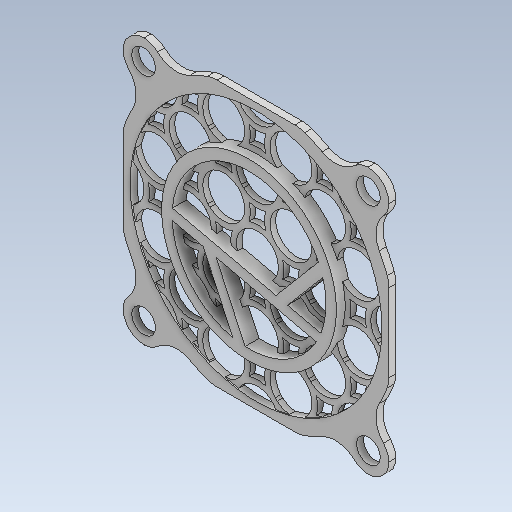
# Autodesk Inventor part: S Fan Cover
Saved by Autodesk Inventor 2022 (Build 260153000, 153)
## iProperties
Created: 2019-12-19
Part Number: S Fan Cover
Material: Generic
Document SubType Name: Modeling
Designer: pepd9
Density: 1 g/cm^3
Appearance: Default
Author: pepd9
Autodesk Inventor part; units mm, degrees
ref_plane "YZ Plane" through (0, 0, 0) normal (1, 0, 0) x (0, 1, 0)
ref_plane "XZ Plane" through (0, 0, 0) normal (0, 1, 0) x (-1, 0, 0)
ref_plane "XY Plane" through (0, 0, 0) normal (0, 0, 1) x (1, 0, 0)
sketch "Sketch1" plane through (0, 0, 0) normal (0, 0, 1) x (1, 0, 0)
  circle A0 centre (1.9624, -34.0934) radius 1.5 projected
  circle A1 centre (1.9624, -1.9624) radius 1.5 projected
  circle A2 centre (34.0934, -1.9624) radius 1.5 projected
  circle A3 centre (34.0934, -34.0934) radius 1.5 projected
  line L0 (1.9624, -34.0934) -> (34.0934, -1.9624)
  line L1 (37.0279, -37.0279) -> (-0.9721, -37.0279)
  line L2 (-0.9721, -37.0279) -> (-0.9721, 0.9721)
  line L3 (-0.9721, 0.9721) -> (37.0279, 0.9721)
  line L4 (37.0279, 0.9721) -> (37.0279, -37.0279)
  line L5 (37.0279, -37.0279) -> (-0.9721, 0.9721) construction
  line L6 (-0.9721, -37.0279) -> (37.0279, 0.9721) construction
  circle A4 centre (1.9624, -34.0934) radius 1.7
  circle A5 centre (34.0934, -34.0934) radius 1.7
  circle A6 centre (34.0934, -1.9624) radius 1.7
  circle A7 centre (1.9624, -1.9624) radius 1.7
  point P0 (0, 0)
  point P1 (18.0279, -18.0279)
  dimension "d0" = 38
  dimension "d1" = 38
  dimension "d5" = 0.2
  dimension "d6" = 0.2
  dimension "d7" = 0.2
  dimension "d8" = 0.2
  constraints: 14 end point, 4 centre point, 3 midpoint, 2 parallel, 1 horizontal, 1 perpendicular
  measures "d0" distance of L2.end L3.end
  measures "d1" distance of L1.end L2.end
  measures "d5" radial gap between concentric circles of A0 A4
  measures "d6" radial gap between concentric circles of A3 A5
  measures "d7" radial gap between concentric circles of A2 A6
  measures "d8" radial gap between concentric circles of A1 A7
extrude "Extrusion1" add sketch "Sketch1" along normal blind 1 contours L1 L2 L3 L4
fillet "Fillet1" radius 3 4 edges at (-0.9721, 0.9721, 0.5) (-0.9721, -37.0279, 0.5) (37.0279, -37.0279, 0.5) (37.0279, 0.9721, 0.5)
sketch "Sketch2" plane through (0, 0, 1) normal (0, 0, 1) x (1, 0, 0)
  arc A0 (37.0279, -2.0279) -> (34.0279, 0.9721) centre (34.0279, -2.0279) ccw projected
  line L0 (34.0279, 0.9721) -> (2.0279, 0.9721) projected
  arc A1 (2.0279, 0.9721) -> (-0.9721, -2.0279) centre (2.0279, -2.0279) ccw projected
  line L1 (-0.9721, -2.0279) -> (-0.9721, -34.0279) projected
  arc A2 (-0.9721, -34.0279) -> (2.0279, -37.0279) centre (2.0279, -34.0279) ccw projected
  line L2 (2.0279, -37.0279) -> (34.0279, -37.0279) projected
  arc A3 (34.0279, -37.0279) -> (37.0279, -34.0279) centre (34.0279, -34.0279) ccw projected
  line L3 (37.0279, -34.0279) -> (37.0279, -2.0279) projected
  circle A4 centre (1.9624, -34.0934) radius 1.7 projected
  circle A5 centre (34.0934, -1.9624) radius 1.7 projected
  circle A6 centre (34.0934, -34.0934) radius 1.7 projected
  circle A7 centre (1.9624, -1.9624) radius 1.7 projected
  circle A8 centre (1.9624, -34.0934) radius 1.7 projected
  line L4 (1.9624, -34.0934) -> (34.0934, -1.9624)
  circle A9 centre (18.0279, -18.0279) radius 18
  point P0 (0, 0)
  dimension "d9" = 36
  constraints: 2 end point, 1 centre point, 1 midpoint
  measures "d9" diameter of A9
extrude "Extrusion2" cut sketch "Sketch2" against normal through all contours A9 L4 | L4 A9
sketch "Sketch3" plane through (0, 0, 1) normal (0, 0, 1) x (1, 0, 0)
  circle A0 centre (18.0279, -18.0279) radius 18 projected
  arc A1 (37.0279, -2.0279) -> (34.0279, 0.9721) centre (34.0279, -2.0279) ccw projected
  line L0 (34.0279, 0.9721) -> (2.0279, 0.9721) projected
  arc A2 (2.0279, 0.9721) -> (-0.9721, -2.0279) centre (2.0279, -2.0279) ccw projected
  line L1 (-0.9721, -2.0279) -> (-0.9721, -34.0279) projected
  arc A3 (-0.9721, -34.0279) -> (2.0279, -37.0279) centre (2.0279, -34.0279) ccw projected
  line L2 (2.0279, -37.0279) -> (34.0279, -37.0279) projected
  arc A4 (34.0279, -37.0279) -> (37.0279, -34.0279) centre (34.0279, -34.0279) ccw projected
  line L3 (37.0279, -34.0279) -> (37.0279, -2.0279) projected
  circle A5 centre (1.9624, -34.0934) radius 1.7 projected
  circle A6 centre (34.0934, -1.9624) radius 1.7 projected
  circle A7 centre (34.0934, -34.0934) radius 1.7 projected
  circle A8 centre (1.9624, -1.9624) radius 1.7 projected
  circle A9 centre (18.0279, -18.0279) radius 20
  circle A10 centre (34.0934, -34.0934) radius 1.7 projected
  arc A11 (34.0279, -37.0279) -> (37.0279, -34.0279) centre (34.0279, -34.0279) ccw projected
  circle A12 centre (34.0934, -34.0934) radius 2.9352
  arc A13 (37.0279, -2.0279) -> (34.0279, 0.9721) centre (34.0279, -2.0279) ccw projected
  circle A14 centre (34.0934, -1.9624) radius 2.9352
  arc A15 (2.0279, 0.9721) -> (-0.9721, -2.0279) centre (2.0279, -2.0279) ccw projected
  circle A16 centre (1.9624, -1.9624) radius 2.9352
  circle A17 centre (1.9624, -34.0934) radius 2.9352
  point P0 (0, 0)
  point P1 (2.0279, -37.0279)
  point P2 (11.7829, -37.0279)
  point P3 (4.6363, -32.8827)
  point P4 (3.1731, -31.4195)
  point P5 (-0.9721, -24.2729)
  point P6 (3.1731, -4.6363)
  point P7 (-0.9721, -11.7829)
  point P8 (4.6363, -3.1731)
  point P9 (11.7829, 0.9721)
  point P10 (31.4195, -3.1731)
  point P11 (24.2729, 0.9721)
  point P12 (32.8827, -4.6363)
  point P13 (37.0279, -11.7829)
  point P14 (31.4195, -32.8827)
  point P15 (24.2729, -37.0279)
  point P16 (32.8827, -31.4195)
  point P17 (37.0279, -24.2729)
  dimension "d12" = 40
  constraints: 5 coincident, 1 centre point, 12 other
  measures "d12" diameter of A9
extrude "Extrusion3" cut sketch "Sketch3" against normal through all contours L3 A9 A14 | A14 A9 L0 | L3 A12 A9 | A9 A16 L0 | A12 L2 A9 | A16 A9 L1 | L2 A17 A9 | A9 A17 L1
fillet "Fillet2" radius 4 16 edges at (32.8827, -31.4195, 0.5) (37.0279, -24.2729, 0.5) (31.4195, -32.8827, 0.5) (32.8827, -4.6363, 0.5) (31.4195, -3.1731, 0.5) (37.0279, -11.7829, 0.5) (24.2729, 0.9721, 0.5) (11.7829, 0.9721, 0.5) (4.6363, -3.1731, 0.5) (3.1731, -4.6363, 0.5) (-0.9721, -11.7829, 0.5) (-0.9721, -24.2729, 0.5) (3.1731, -31.4195, 0.5) (4.6363, -32.8827, 0.5) (11.7829, -37.0279, 0.5) (24.2729, -37.0279, 0.5)
sketch "Sketch4" plane through (0, 0, 0) normal (0, 0, -1) x (-1, 0, 0)
  circle A0 centre (-18.0279, -18.0279) radius 18 projected
  circle A1 centre (-18.0279, -18.0279) radius 12.5
  circle A2 centre (-18.0279, -18.0279) radius 11
  line L0 (-6.2121, -18.41) -> (-28.6137, -23.5698)
  line L1 (-6.6166, -16.9639) -> (-29.0182, -22.1237)
  line L2 (-17.5588, -29.2308) -> (-13.3321, -20.05)
  line L3 (-16.1962, -29.8581) -> (-11.4849, -19.6245)
  line L4 (-21.8908, -20.4821) -> (-27.9649, -13.3103)
  line L5 (-23.5356, -20.8609) -> (-28.5765, -14.9091)
  point P0 (0, 0)
  point P1 (-7.0429, -18.6014)
  point P2 (-15.6992, -28.7786)
  point P3 (-28.3016, -21.9587)
  point P4 (-7.0698, -17.0683)
  point P5 (-17.4586, -29.0132)
  point P6 (-27.6552, -23.3491)
  dimension "d18" = 25
  dimension "d19" = 22
  dimension "d20" = 1.5
  dimension "d22" = 1.5
  dimension "d23" = 1.5
  constraints: 12 end point, 4 point on line, 3 parallel, 2 centre point, 2 coincident, 2 point on circle
  measures "d18" diameter of A1
  measures "d19" diameter of A2
  measures "d20" distance between parallel lines of L0 L1
  measures "d22" distance between parallel lines of L2 L3
  measures "d23" distance between parallel lines of L4 L5
extrude "Extrusion4" add sketch "Sketch4" against normal blind 2 contours A1 | L4 L1 L5 A2 | A2 L0 L1 | L2 L0 L3 A2
sketch "Sketch5" plane through (0, 0, 0) normal (0, 0, -1) x (-1, 0, 0)
  arc A0 (-7.0698, -17.0683) -> (-27.9649, -13.3103) centre (-18.0279, -18.0279) ccw projected
  circle A1 centre (-18.0279, -18.0279) radius 3
  circle A2 centre (-18.0279, -18.0279) radius 3.8
  line L0 (-18.0279, -18.0279) -> (-18.0279, -16.2513)
  line L1 (-18.0279, -18.0279) -> (-19.9201, -16.1357)
  line L2 (-18.0279, -18.0279) -> (-15.352, -18.0279) construction
  circle A3 centre (-22.8362, -13.2196) radius 3
  circle A4 centre (-22.8362, -13.2196) radius 3.8
  circle A5 centre (-27.6446, -8.4112) radius 3
  circle A6 centre (-27.6446, -8.4112) radius 3.8
  circle A7 centre (-13.2196, -22.8362) radius 3
  circle A8 centre (-13.2196, -22.8362) radius 3.8
  circle A9 centre (-8.4112, -27.6446) radius 3
  circle A10 centre (-8.4112, -27.6446) radius 3.8
  circle A11 centre (-27.6446, -27.6446) radius 3.8
  circle A12 centre (-27.6446, -27.6446) radius 3
  circle A13 centre (-22.8362, -22.8362) radius 3
  circle A14 centre (-22.8362, -22.8362) radius 3.8
  circle A15 centre (-13.2196, -13.2196) radius 3.8
  circle A16 centre (-13.2196, -13.2196) radius 3
  circle A17 centre (-8.4112, -8.4112) radius 3
  circle A18 centre (-8.4112, -8.4112) radius 3.8
  circle A19 centre (-18.0279, -8.4279) radius 3.8
  circle A20 centre (-18.0279, -8.4279) radius 3
  circle A21 centre (-13.2196, -3.6196) radius 3.8
  circle A22 centre (-13.2196, -3.6196) radius 3
  circle A23 centre (-22.8362, -3.6196) radius 3
  circle A24 centre (-22.8362, -3.6196) radius 3.8
  circle A25 centre (-32.4362, -13.2196) radius 3
  circle A26 centre (-32.4362, -13.2196) radius 3.8
  circle A27 centre (-32.4362, -22.8362) radius 3.8
  circle A28 centre (-32.4362, -22.8362) radius 3
  circle A29 centre (-27.6279, -18.0279) radius 3
  circle A30 centre (-27.6279, -18.0279) radius 3.8
  circle A31 centre (-22.8362, -32.4362) radius 3
  circle A32 centre (-22.8362, -32.4362) radius 3.8
  circle A33 centre (-13.2196, -32.4362) radius 3.8
  circle A34 centre (-13.2196, -32.4362) radius 3
  circle A35 centre (-18.0279, -27.6279) radius 3
  circle A36 centre (-18.0279, -27.6279) radius 3.8
  circle A37 centre (-3.6196, -22.8362) radius 3
  circle A38 centre (-3.6196, -22.8362) radius 3.8
  circle A39 centre (-3.6196, -13.2196) radius 3.8
  circle A40 centre (-3.6196, -13.2196) radius 3
  circle A41 centre (-8.4279, -18.0279) radius 3
  circle A42 centre (-8.4279, -18.0279) radius 3.8
  circle A43 centre (-18.0279, 1.1721) radius 3
  circle A44 centre (-18.0279, 1.1721) radius 3.8
  circle A45 centre (-37.2279, -18.0279) radius 3
  circle A46 centre (-37.2279, -18.0279) radius 3.8
  circle A47 centre (-18.0279, -37.2279) radius 3
  circle A48 centre (-18.0279, -37.2279) radius 3.8
  circle A49 centre (1.1721, -18.0279) radius 3
  circle A50 centre (1.1721, -18.0279) radius 3.8
  circle A51 centre (-18.0279, -18.0279) radius 18 projected
  circle A52 centre (-27.6446, 1.1888) radius 3
  circle A53 centre (-27.6446, 1.1888) radius 3.8
  circle A54 centre (-32.4529, -3.6029) radius 3
  circle A55 centre (-32.4529, -3.6029) radius 3.8
  circle A56 centre (-37.2446, -8.4112) radius 3.8
  circle A57 centre (-37.2446, -8.4112) radius 3
  circle A58 centre (-37.2446, -27.6446) radius 3
  circle A59 centre (-37.2446, -27.6446) radius 3.8
  circle A60 centre (-32.4529, -32.4529) radius 3
  circle A61 centre (-32.4529, -32.4529) radius 3.8
  circle A62 centre (-27.6446, -37.2446) radius 3
  circle A63 centre (-27.6446, -37.2446) radius 3.8
  circle A64 centre (-8.4112, -37.2446) radius 3
  circle A65 centre (-8.4112, -37.2446) radius 3.8
  circle A66 centre (-3.6029, -32.4529) radius 3
  circle A67 centre (-3.6029, -32.4529) radius 3.8
  circle A68 centre (1.1888, -27.6446) radius 3
  circle A69 centre (1.1888, -27.6446) radius 3.8
  circle A70 centre (1.1888, -8.4112) radius 3
  circle A71 centre (1.1888, -8.4112) radius 3.8
  circle A72 centre (-3.6029, -3.6029) radius 3
  circle A73 centre (-3.6029, -3.6029) radius 3.8
  circle A74 centre (-8.4112, 1.1888) radius 3
  circle A75 centre (-8.4112, 1.1888) radius 3.8
  point P0 (0, 0)
  point P1 (-22.6315, -35.4292)
  point P2 (-24.7974, -34.7065)
  point P3 (-26.4404, -12.0154)
  point P4 (-26.4425, -14.4175)
  point P5 (-28.8321, -14.4237)
  point P6 (-28.83, -12.0216)
  point P7 (-24.0404, -9.6154)
  point P8 (-23.8554, -8.6984)
  point P9 (-21.7532, -7.6779)
  point P10 (-21.6383, -9.6133)
  point P11 (-19.2321, -14.4237)
  point P12 (-19.2259, -12.0341)
  point P13 (-16.8299, -12.0341)
  point P14 (-16.8237, -14.4237)
  point P15 (-16.8237, -21.6321)
  point P16 (-16.8299, -24.0217)
  point P17 (-19.2259, -24.0217)
  point P18 (-19.2321, -21.6321)
  point P19 (-14.4237, -19.2321)
  point P20 (-14.4237, -16.8237)
  point P21 (-12.0341, -16.8299)
  point P22 (-12.0341, -19.2259)
  point P23 (-11.258, -9.358)
  point P24 (-10.6717, -6.4389)
  point P25 (-10.3915, -6.1576)
  point P26 (-6.1576, -10.3915)
  point P27 (-6.4389, -10.6717)
  point P28 (-9.358, -11.258)
  point P29 (-12.0154, -9.6154)
  point P30 (-14.4175, -9.6133)
  point P31 (-14.4237, -7.2237)
  point P32 (-12.0216, -7.2258)
  point P33 (-26.6978, -11.258)
  point P34 (-29.6169, -10.6717)
  point P35 (-29.8982, -10.3915)
  point P36 (-25.6643, -6.1576)
  point P37 (-25.3841, -6.4389)
  point P38 (-24.7978, -9.358)
  point P39 (-11.2394, -5.8732)
  point P40 (-13.4243, -0.6266)
  point P41 (-15.373, -0.2248)
  point P42 (-20.0081, -1.0815)
  point P43 (-20.2884, -0.8003)
  point P44 (-20.6828, -0.2248)
  point P45 (-21.0248, -0.2791)
  point P46 (-26.2908, -2.0365)
  point P47 (-27.2919, -2.5948)
  point P48 (-26.4404, -2.4154)
  point P49 (-26.4466, -4.805)
  point P50 (-28.8487, -4.8071)
  point P51 (-28.6543, -3.4993)
  point P52 (-29.5054, -4.1619)
  point P53 (-31.8939, -6.5504)
  point P54 (-32.5565, -7.4015)
  point P55 (-31.2487, -7.2071)
  point P56 (-31.2508, -9.6092)
  point P57 (-33.6404, -9.6154)
  point P58 (-33.461, -8.7639)
  point P59 (-34.0193, -9.765)
  point P60 (-36.0425, -14.4175)
  point P61 (-36.0425, -21.6383)
  point P62 (-34.0193, -26.2908)
  point P63 (-33.461, -27.2919)
  point P64 (-33.6404, -26.4404)
  point P65 (-31.2508, -26.4466)
  point P66 (-31.2487, -28.8487)
  point P67 (-32.5565, -28.6543)
  point P68 (-31.8939, -29.5054)
  point P69 (-29.5054, -31.8939)
  point P70 (-28.6543, -32.5565)
  point P71 (-28.8487, -31.2487)
  point P72 (-26.4466, -31.2508)
  point P73 (-26.4404, -33.6404)
  point P74 (-27.2919, -33.461)
  point P75 (-24.8275, -34.6942)
  point P76 (-24.9575, -34.5575)
  point P77 (-25.0967, -30.4638)
  point P78 (-24.8164, -30.1826)
  point P79 (-20.5758, -34.4086)
  point P80 (-20.856, -34.6898)
  point P81 (-20.6828, -35.831)
  point P82 (-15.373, -35.831)
  point P83 (-13.4243, -35.4292)
  point P84 (-11.0983, -34.5575)
  point P85 (-11.2283, -34.6942)
  point P86 (-8.7639, -33.461)
  point P87 (-9.6154, -33.6404)
  point P88 (-9.6092, -31.2508)
  point P89 (-7.2071, -31.2487)
  point P90 (-7.4015, -32.5565)
  point P91 (-6.5504, -31.8939)
  point P92 (-4.1619, -29.5054)
  point P93 (-3.4993, -28.6543)
  point P94 (-4.8071, -28.8487)
  point P95 (-4.805, -26.4466)
  point P96 (-2.4154, -26.4404)
  point P97 (-2.5948, -27.2919)
  point P98 (-1.3493, -24.7974)
  point P99 (-0.6266, -22.6315)
  point P100 (-0.2248, -20.6828)
  point P101 (-0.2248, -15.373)
  point P102 (-0.6266, -13.4243)
  point P103 (-5.8732, -11.2394)
  point P104 (-5.592, -10.9591)
  point P105 (-1.3493, -11.2584)
  point P106 (-2.5948, -8.7639)
  point P107 (-2.4154, -9.6154)
  point P108 (-4.805, -9.6092)
  point P109 (-4.8071, -7.2071)
  point P110 (-3.4993, -7.4015)
  point P111 (-4.1619, -6.5504)
  point P112 (-6.5504, -4.1619)
  point P113 (-7.4015, -3.4993)
  point P114 (-7.2071, -4.8071)
  point P115 (-9.6092, -4.805)
  point P116 (-9.6154, -2.4154)
  point P117 (-8.7639, -2.5948)
  point P118 (-11.2283, -1.3616)
  point P119 (-11.0983, -1.4983)
  point P120 (-10.9591, -5.592)
  point P121 (-25.0967, -5.592)
  point P122 (-24.7974, -1.3493)
  point P123 (-22.6315, -0.6266)
  point P124 (-20.856, -1.366)
  point P125 (-20.5758, -1.6472)
  point P126 (-24.8164, -5.8732)
  point P127 (-26.4404, -24.0404)
  point P128 (-28.83, -24.0342)
  point P129 (-28.8321, -21.6321)
  point P130 (-26.4425, -21.6383)
  point P131 (-25.6555, -15.7674)
  point P132 (-25.3743, -16.0477)
  point P133 (-25.3743, -20.0081)
  point P134 (-25.6555, -20.2884)
  point P135 (-25.0898, -20.856)
  point P136 (-24.8086, -20.5758)
  point P137 (-20.5758, -24.8086)
  point P138 (-20.856, -25.0898)
  point P139 (-30.1826, -11.2394)
  point P140 (-34.4086, -15.48)
  point P141 (-34.6898, -15.1998)
  point P142 (-35.4292, -13.4243)
  point P143 (-34.7065, -11.2584)
  point P144 (-30.4638, -10.9591)
  point P145 (-12.0154, -26.4404)
  point P146 (-12.0216, -28.83)
  point P147 (-14.4237, -28.8321)
  point P148 (-14.4175, -26.4425)
  point P149 (-30.4638, -25.0967)
  point P150 (-34.7065, -24.7974)
  point P151 (-35.4292, -22.6315)
  point P152 (-34.6898, -20.856)
  point P153 (-34.4086, -20.5758)
  point P154 (-30.1826, -24.8164)
  point P155 (-35.2555, -20.2884)
  point P156 (-35.831, -20.6828)
  point P157 (-35.831, -15.373)
  point P158 (-35.2555, -15.7674)
  point P159 (-34.9743, -16.0477)
  point P160 (-34.9743, -20.0081)
  point P161 (-24.0342, -28.83)
  point P162 (-24.0404, -26.4404)
  point P163 (-21.6383, -26.4425)
  point P164 (-21.6321, -28.8321)
  point P165 (-16.8237, -31.2321)
  point P166 (-16.8299, -33.6217)
  point P167 (-19.2259, -33.6217)
  point P168 (-19.2321, -31.2321)
  point P169 (-11.2472, -20.5758)
  point P170 (-10.966, -20.856)
  point P171 (-15.1998, -25.0898)
  point P172 (-15.48, -24.8086)
  point P173 (-4.8237, -16.8237)
  point P174 (-2.4341, -16.8299)
  point P175 (-2.4341, -19.2259)
  point P176 (-4.8237, -19.2321)
  point P177 (-10.4003, -20.2884)
  point P178 (-10.6815, -20.0081)
  point P179 (-10.6815, -16.0477)
  point P180 (-10.4003, -15.7674)
  point P181 (-9.6154, -24.0404)
  point P182 (-9.6133, -21.6383)
  point P183 (-7.2237, -21.6321)
  point P184 (-7.2258, -24.0342)
  point P185 (-15.7674, -25.6555)
  point P186 (-20.2884, -25.6555)
  point P187 (-20.0081, -25.3743)
  point P188 (-16.0477, -25.3743)
  point P189 (-31.2321, -16.8237)
  point P190 (-31.2321, -19.2321)
  point P191 (-33.6217, -19.2259)
  point P192 (-33.6217, -16.8299)
  point P193 (-25.3841, -29.6169)
  point P194 (-25.6643, -29.8982)
  point P195 (-29.8982, -25.6643)
  point P196 (-29.6169, -25.3841)
  point P197 (-16.8237, -4.8237)
  point P198 (-19.2321, -4.8237)
  point P199 (-19.2259, -2.4341)
  dimension "d26" = 6
  dimension "d27" = 0.8
  dimension "d28" = 135
  dimension "d31" = 6.8
  dimension "d38" = 6.8
  dimension "d45" = 90
  dimension "d49" = 9.6
  dimension "d56" = 9.6
  dimension "d63" = 360
  dimension "d67" = 19.2
  dimension "d74" = 360
  dimension "d78" = 6.8
  dimension "d85" = 360
  constraints: 74 centre point, 6 end point, 4 vertical, 1 coincident, 1 equal length, 1 horizontal, 137 other
  measures "d26" diameter of A1
  measures "d27" radial gap between concentric circles of A1 A2
  measures "d28" angle of L2 L1
  measures "d31" distance of A1.centre A3.centre
  measures "d38" distance of A1.centre A7.centre
  measures "d49" distance of A1.centre A19.centre
  measures "d56" distance of A15.centre A21.centre
  measures "d67" distance of A1.centre A43.centre
  measures "d78" distance of A23.centre A52.centre
extrude "Extrusion5" add sketch "Sketch5" against normal blind 0.8 contours A41 A15 A42 A0 | A0 A42 A39 A41 | A39 A42 | A39 A42 A38 A41 | A41 A15 A42 A16 | A15 A41 | A18 A15 A17 A0 | A0 A17 A39 A18 | A39 A18 A40 A42 | A42 A16 A18 A15 | A42 A40 A50 A39 | A41 A8 A42 A15 | A17 A0 | A18 A15 | A39 A17 A18 A40 | A16 A42 | A50 A40 A51 A39 A49 | A39 A49 A38 A50 | A38 A42 | A38 A42 A8 A41 | A15 A2 A16 A42 | A41 A8 A42 A7 | A8 A41 | A17 A15 A18 A0 | A0 A18 A21 A17 | A39 A17 | A16 A19 A15 A18 | A40 A18 | A50 A37 A42 A38 | A38 A49 A51 A50 A37 | A42 A37 A10 A38 | A15 A2 | A2 A8 A1 A15 | A42 A7 A2 A8 | A21 A18 A22 A17 | A17 A21 | A17 A73 A18 A39 | A19 A16 | A16 A19 A15 A20 | A18 A39 A71 A40 | A40 A51 A50 | A2 A15 A19 A16 | A39 A51 A49 | A38 A9 A8 A10 | A10 A37 A38 A9 | A8 A10 A7 A42 | A1 A4 A2 A15 | A2 A8 | A7 A42 | A19 A15 A20 A0 | A0 A20 A21 A19 | A21 A19 A22 A18 | A21 A18 A73 A17 | A71 A51 A40 | A71 A39 A51 | A49 A51 A38 | A50 A51 A37 | A8 A10 | A1 A14 A2 A4 | A4 A2 | A7 A36 A8 A2 | A8 A2 A14 A1 | A0 A20 | A21 A19 | A18 A22 | A73 A18 | A18 A22 A75 A21 | A20 A15 | A71 A51 A39 | A19 A4 A20 A15 | A2 A3 A19 A4 | A37 A69 A38 A10 | A9 A33 A10 A8 | A10 A8 A36 A7 | A38 A10 A67 A9 | A14 A2 | A4 A30 A3 A2 | A36 A7 | A7 A36 A8 A35 | A20 A4 A19 A0 | A0 A19 A24 A20 | A20 A24 A19 A21 | A19 A21 A44 A22 | A73 A51 A72 A18 | A18 A72 A51 A73 | A19 A3 A4 A20 | A51 A69 A37 | A69 A51 A38 | A9 A33 A10 A34 | A14 A36 A13 A2 | A2 A13 A30 A14 | A30 A14 A29 A4 | A4 A29 A30 A3 | A8 A35 A14 A36 | A0 A6 A24 A19 | A24 A19 | A4 A20 | A44 A21 A43 A51 A22 | A75 A51 A21 | A21 A51 A75 | A19 A3 | A3 A30 | A38 A51 A69 | A36 A33 A35 A8 | A10 A34 A36 A33 | A9 A67 A10 A33 | A67 A10 | A30 A13 A14 A29 | A4 A29 | A35 A8 | A14 A35 A36 A13 | A6 A4 A5 A0 | A0 A5 A24 A6 | A24 A6 A23 A19 | A19 A3 A6 A4 | A19 A23 A44 A24 | A44 A24 A43 A21 | A44 A51 A22 | A30 A4 A6 A3 | A67 A51 A66 A10 | A36 A33 | A33 A65 A34 A10 | A10 A66 A51 A67 | A30 A13 | A29 A14 | A29 A26 A30 A4 | A14 A35 | A13 A36 | A5 A0 | A6 A4 | A24 A5 A6 A23 | A44 A23 A51 A24 A43 | A34 A48 A33 A36 | A33 A36 A32 A35 | A13 A11 A14 A30 | A14 A30 A27 A29 | A29 A27 A30 A26 | A26 A30 | A35 A32 A36 A14 | A36 A14 A11 A13 | A5 A4 A6 A0 | A0 A6 A26 A5 | A23 A6 | A24 A5 | A43 A51 A21 | A43 A24 | A44 A23 | A30 A25 A6 A26 | A34 A48 A51 A33 A47 | A32 A36 | A65 A51 A33 | A33 A51 A65 | A11 A14 | A27 A30 | A26 A46 A25 A30 | A26 A6 A25 A5 | A5 A26 | A6 A24 A53 A23 | A5 A55 A6 A24 | A24 A51 A43 | A23 A51 A44 | A34 A51 A48 | A33 A47 A32 A48 | A32 A48 A31 A36 | A36 A31 A11 A32 | A11 A32 A12 A14 | A14 A12 A27 A11 | A27 A11 A28 A30 | A30 A28 A46 A27 | A46 A27 A45 A26 | A26 A45 A51 A46 A25 | A26 A6 A55 A5 | A53 A51 A23 | A53 A24 A51 | A55 A6 | A51 A44 A24 | A51 A23 | A23 A51 A53 A24 A44 | A25 A46 | A32 A47 A51 A48 A31 | A11 A31 A32 A12 | A27 A12 A11 A28 | A46 A28 A51 A27 A45 | A26 A45 | A6 A25 | A6 A25 A56 A26 | A6 A54 A51 A55 | A53 A51 A24 | A51 A24 A53 | A55 A51 A54 A6 | A46 A51 A25 | A51 A47 A33 | A31 A48 | A11 A31 | A12 A32 | A27 A12 | A28 A11 | A46 A28 | A45 A27 | A45 A51 A26 | A56 A51 A26 | A26 A51 A56 | A51 A46 A26 A56 A25 | A25 A51 | A51 A26 A46 | A47 A51 A32 | A48 A51 A31 | A31 A63 A32 A11 | A32 A11 A61 A12 | A12 A61 A11 A27 | A11 A27 A59 A28 | A28 A51 A46 | A27 A51 A45 | A25 A51 A56 | A51 A56 A26 | A31 A51 | A63 A51 A32 | A61 A11 | A59 A51 A28 | A59 A27 A51 | A51 A28 | A28 A51 A59 A27 A46 | A46 A27 A51 | A61 A51 A60 A11 | A32 A51 A63 | A11 A60 A51 A61 | A59 A51 A27 | A51 A27 A59 picked at (-1.9546, -10.3515) picked at (-2.3713, -9.2859) picked at (-1.9546, -25.7043) picked at (-10.3515, -1.9546) picked at (-9.2859, -2.3713) picked at (-2.3713, -26.7699) picked at (-9.2859, -33.6845) picked at (-10.3515, -34.1012) picked at (-25.7043, -34.1012) picked at (-26.7699, -33.6845)
body "Solid1"
